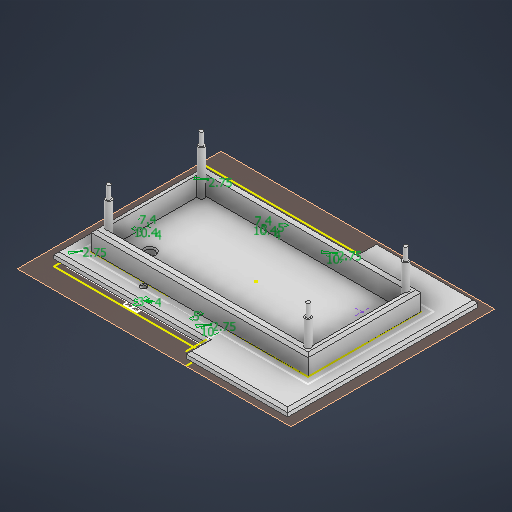
# Autodesk Inventor part: bot-buggy-body-assembly-ready-group2
Saved by Autodesk Inventor 2026.2 (Build 302298010, 298A)
## iProperties
Created: 2026-02-09
Part Number: bot-buggy-body-assembly-ready-group2
Material: Generic
Document SubType Name: Modeling
Designer: dm2166
Density: 1 g/cm^3
Appearance: Default
Mass: 226.605 g
Surface Area: 796.438 cm^2
Volume: 226.605 cm^3
Author: dm2166
Autodesk Inventor part; units mm, degrees
ref_plane "YZ Plane" through (0, 0, 0) normal (1, 0, 0) x (0, 1, 0)
ref_plane "XZ Plane" through (0, 0, 0) normal (0, 1, 0) x (-1, 0, 0)
ref_plane "XY Plane" through (0, 0, 0) normal (0, 0, 1) x (1, 0, 0)
sketch "Sketch1" plane through (0, 0, 0) normal (0, 1, 0) x (-1, 0, 0)
  line L0 (-85.5, -44.5) -> (85.5, -44.5)
  line L1 (85.5, -44.5) -> (85.5, 44.5)
  line L2 (85.5, 44.5) -> (-85.5, 44.5)
  line L3 (-85.5, 44.5) -> (-85.5, -44.5)
  line L4 (-85.5, -44.5) -> (85.5, 44.5) construction
  line L5 (85.5, -44.5) -> (-85.5, 44.5) construction
  line L6 (-81, -38.5) -> (81, -38.5)
  line L7 (81, -38.5) -> (81, 38.5)
  line L8 (81, 38.5) -> (-81, 38.5)
  line L9 (-81, 38.5) -> (-81, -38.5)
  line L10 (-81, -38.5) -> (81, 38.5) construction
  line L11 (81, -38.5) -> (-81, 38.5) construction
  line L12 (81, 38.5) -> (79.55, 38.5)
  line L13 (81, 37.05) -> (81, 38.5)
  circle A0 centre (79.55, 36.5) radius 1.45
  circle A1 centre (79.55, -36.5) radius 1.45
  circle A2 centre (-79.55, -38.5) radius 1.45
  circle A3 centre (-79.55, 38.4727) radius 1.45
  line L14 (81, -38.5) -> (81, -35.6)
  line L15 (-81, -38.5) -> (-78.1, -38.5)
  line L16 (-81, 38.5) -> (-81, 35.6)
  circle A4 centre (-79.55, 38.4727) radius 2.5
  line L17 (-95.5566, 0) -> (75.4434, 0)
  line L18 (0, 31.9167) -> (0, -57.0833)
  circle A5 centre (-79.55, -38.5) radius 2.5
  circle A6 centre (79.55, 36.5) radius 2.5
  circle A7 centre (79.55, -36.5) radius 2.5
  line L19 (140, 0) -> (-140, 0) projected
  line L20 (0, -105) -> (0, 105) projected
  line L21 (-100, 59.2475) -> (100, 59.2475)
  line L22 (100, 59.2475) -> (100, -59.2475)
  line L23 (100, -59.2475) -> (-100, -59.2475)
  line L24 (-100, -59.2475) -> (-100, 59.2475)
  line L25 (-100, 59.2475) -> (100, -59.2475) construction
  line L26 (100, 59.2475) -> (-100, -59.2475) construction
  line L27 (-100, 75) -> (-20, 75)
  line L28 (-20, 75) -> (-20, -75)
  line L29 (-20, -75) -> (-100, -75)
  line L30 (-100, -75) -> (-100, 75)
  line L31 (-100, 75) -> (-20, -75) construction
  line L32 (-20, 75) -> (-100, -75) construction
  line L33 (-79.55, 38.5) -> (-79.55, -38.5)
  line L34 (79.55, 36.5) -> (79.55, -36.5)
  line L35 (-96.0841, 75) -> (-26.0841, 75)
  line L36 (-26.0841, -75) -> (-94.0841, -75)
  point P0 (0, 0)
  point P1 (-80.9997, 38.5)
  point P2 (-81, 38.4727)
  point P3 (-81, -38.5)
  point P4 (-81, -38.5)
  point P5 (79.55, -38.5)
  point P6 (81, -36.5)
  point P7 (81, 36.5)
  point P8 (-60, 0)
  point P9 (-20, 59.2475)
  point P10 (-20, -59.2475)
  point P11 (-79.55, 0)
  point P12 (-78.1003, 38.5)
  point P13 (79.55, 0)
  dimension "d0" = 171
  dimension "d1" = 89
  dimension "d2" = 162
  dimension "d3" = 77
  dimension "d7" = 2.9
  dimension "d8" = 2.9
  dimension "d9" = 2.9
  dimension "d10" = 2.9
  dimension "d53" = 5
  dimension "d56" = 200
  dimension "d57" = 80
  dimension "d58" = 150
  dimension "d82" = 77
  dimension "d84" = 36.5
  dimension "d85" = 36.5
  constraints: 70 end point, 11 parallel, 10 midpoint, 8 centre point, 7 horizontal, 6 perpendicular, 5 point on line, 3 collinear, 3 concentric, 1 vertical, 4 other
  measures "d0" distance of L2.end L1.end
  measures "d1" distance of L1.end L0.end
  measures "d2" distance of L8.end L7.end
  measures "d3" distance of L7.end L6.end
  measures "d7" diameter of A0
  measures "d8" diameter of A1
  measures "d9" diameter of A2
  measures "d10" diameter of A3
  measures "d53" diameter of A4
  measures "d56" distance of L22.end L23.end
  measures "d57" distance of L28.end L29.end
  measures "d58" distance of L27.end L28.end
  measures "d82" distance of L33.start L33.end
  measures "d84" distance of point (79.55, 0) A1.centre
  measures "d85" distance from line of L19 A0.centre
extrude "Extrusion1" add sketch "Sketch1" along normal blind 55 contours A2 L6 | L6 L33 A2 | L8 L33 A3 | A3 L8 | A2 L33 L6 | L33 L8 A3 | A1 | A0
extrude "Extrusion2" add sketch "Sketch1" along normal blind 10 contours L28 L17 L18 L6 | L6 A5 L33 L17 L28 | L17 L33 A5 L9 | L9 A4 L33 L17 | L18 L17 L19 L34 A7 L6 | L6 A2 L33 A5 | L28 L8 L20 L18 L17 | L17 L33 A4 L8 L28 | A5 L33 A2 L9 | A7 L34 A1 L7 L6 | L18 L20 L8 A6 L34 L19 L17 | L6 L33 A2 | L8 L33 A3 | L9 A3 L33 A4 | A2 L33 L6 | L33 A3 L8 A4 | L19 L34 A6 L7 | L7 A7 L34 L19 | A7 L7 A1 L34 | L33 L8 A3 | A6 L34 A0 L7 | A1 | L8 L7 A0 L34 A6 | A0
extrude "Extrusion3" add sketch "Sketch1" along normal blind 25 contours L3 L17 L9 A5 L6 L28 L0 | L28 L6 L18 L0 | L3 L2 L28 L8 A4 L9 L17 | L18 L6 A7 L7 L19 L1 L0 | A5 L9 A2 L6 | L2 L20 L8 L28 | L19 L7 A6 L8 L20 L2 L1 | L6 L7 A7 | A2 L6 | A4 L8 A3 L9 | A3 L8 | L7 L8 A6
chamfer "Chamfer1" distance 2 angle 45 4 edges at (0, 25, 44.5) (85.5, 25, 0) (0, 25, -44.5) (-85.5, 25, 0)
extrude "Extrusion11" add sketch "Sketch1" along normal blind 45 contours A5 L9 A2 L6 | L6 A2 L33 A5 | A5 L33 A2 L9 | A7 L34 A1 L7 L6 | L6 L7 A7 | A2 L6 | L6 L33 A2 | L8 L33 A3 | A4 L8 A3 L9 | A3 L8 | L9 A3 L33 A4 | A2 L33 L6 | L33 A3 L8 A4 | A7 L7 A1 L34 | L33 L8 A3 | A6 L34 A0 L7 | L7 L8 A6 | A1 | L8 L7 A0 L34 A6 | A0
extrude "Extrusion12" add sketch "Sketch1" along normal blind 10 contours L0 L28 L23 L24 L19 L17 L3 | L0 L18 L20 L23 L28 | L17 L19 L24 L21 L28 L2 L3 | L0 L1 L19 L22 L23 L20 L18 | L28 L29 L30 L23 | L28 L21 L20 L2 | L1 L2 L20 L21 L22 L19 | L21 L30 L27 L28
chamfer "Chamfer2" distance 2 angle 45 8 edges at (100, 10, 0) (60, 10, 75) (20, 10, 67.1238) (60, 10, -75) (20, 10, -67.1238) (-40, 10, -59.2475) (-40, 10, 59.2475) (-100, 10, 0)
sketch "Sketch4" plane through (0, 0, 0) normal (0, -1, 0) x (1, 0, 0)
  circle A0 centre (-11.2675, 0) radius 2 projected
  circle A1 centre (-71.2675, 0) radius 2 projected
  circle A2 centre (-41.2675, 30) radius 2 projected
  circle A3 centre (-11.2675, 0) radius 1.9
  circle A4 centre (-71.2675, 0) radius 1.9
  circle A5 centre (-41.2675, 30) radius 1.9
  point P0 (0, 0)
  dimension "d64" = 3.8
  constraints: 3 centre point, 3 coincident, 2 equal radius
  measures "d64" diameter of A5
extrude "Extrusion13" add sketch "Sketch4" along normal blind 10 contours A3 | A4 | A5
sketch "Sketch7" plane through (0, 0, 0) normal (0, -1, 0) x (1, 0, 0)
  line L0 (20, -59.2475) -> (-100, -59.2475) projected
  line L1 (20, -75) -> (20, -59.2475) projected
  line L2 (100, -75) -> (20, -75) projected
  line L3 (100, 75) -> (100, -75) projected
  line L4 (20, 75) -> (100, 75) projected
  line L5 (20, 59.2475) -> (20, 75) projected
  line L6 (-100, 59.2475) -> (20, 59.2475) projected
  line L7 (-100, -59.2475) -> (-100, 59.2475) projected
  line L8 (-95, -54.2475) -> (25, -54.2475)
  line L9 (25, -54.2475) -> (25, -70)
  line L10 (25, -70) -> (95, -70)
  line L11 (95, -70) -> (95, 70)
  line L12 (95, 70) -> (25, 70)
  line L13 (25, 70) -> (25, 54.2475)
  line L14 (25, 54.2475) -> (-95, 54.2475)
  line L15 (-95, 54.2475) -> (-95, -54.2475)
  line L16 (-90, -49.2475) -> (30, -49.2475)
  line L17 (30, -49.2475) -> (30, -65)
  line L18 (30, -65) -> (90, -65)
  line L19 (90, -65) -> (90, 65)
  line L20 (90, 65) -> (30, 65)
  line L21 (30, 65) -> (30, 49.2475)
  line L22 (30, 49.2475) -> (-90, 49.2475)
  line L23 (-90, 49.2475) -> (-90, -49.2475)
  circle A0 centre (25, -70) radius 2
  circle A1 centre (25, 70) radius 2
  circle A2 centre (-41.2675, 0) radius 44 projected
  line L24 (-41.2675, -59.2475) -> (-41.2675, 59.2475)
  line L25 (17.4651, 0) -> (-100, 0)
  point P0 (0, 0)
  dimension "d86" = 5
  dimension "d87" = 10
  dimension "d88" = 4
  dimension "d89" = 4
  constraints: 36 end point, 3 midpoint, 2 centre point, 2 coincident, 1 perpendicular, 1 point on line, 14 other
  measures "d86" distance between parallel lines of L0 L8
  measures "d87" distance between parallel lines of L0 L16
  measures "d88" diameter of A0
  measures "d89" diameter of A1
extrude "Extrusion15" add sketch "Sketch7" along normal blind 10 contours A0 L10 L9 | L9 L10 A0 | A1 L12 L13 | L13 L12 A1
fillet "Fillet16" radius 1 1 edges at (23, -10, -70)
fillet "Fillet17" radius 1 1 edges at (23, 0, -70)
fillet "Fillet18" radius 1 1 edges at (23, 0, 70)
fillet "Fillet19" radius 1 1 edges at (23, -10, 70)
sketch "Sketch9" plane through (0, 0, 0) normal (0, -1, 0) x (1, 0, 0)
  line L0 (-100, 59.2475) -> (20, 59.2475) projected
  line L1 (20, -75) -> (20, 75) projected
  line L2 (20, -59.2475) -> (-100, -59.2475) projected
  line L3 (-100, -59.2475) -> (-100, 59.2475) projected
  circle A0 centre (-41.2675, 0) radius 44 projected
  line L4 (-41.2675, -59.2475) -> (-41.2675, 59.2475)
  line L5 (17.4651, 0) -> (-100, 0)
  line L6 (20, -54.2475) -> (-95, -54.2475)
  line L7 (-95, -54.2475) -> (-95, 54.2475)
  line L8 (-95, 54.2475) -> (20, 54.2475)
  line L9 (-36.0675, -57.9475) -> (-46.4675, -57.9475)
  line L10 (-46.4675, -57.9475) -> (-46.4675, -50.5475)
  line L11 (-46.4675, -50.5475) -> (-36.0675, -50.5475)
  line L12 (-36.0675, -50.5475) -> (-36.0675, -57.9475)
  line L13 (-36.0675, -57.9475) -> (-46.4675, -50.5475) construction
  line L14 (-46.4675, -57.9475) -> (-36.0675, -50.5475) construction
  line L15 (-36.0675, 57.9475) -> (-46.4675, 57.9475)
  line L16 (-46.4675, 57.9475) -> (-46.4675, 50.5475)
  line L17 (-46.4675, 50.5475) -> (-36.0675, 50.5475)
  line L18 (-36.0675, 50.5475) -> (-36.0675, 57.9475)
  line L19 (-36.0675, 57.9475) -> (-46.4675, 50.5475) construction
  line L20 (-46.4675, 57.9475) -> (-36.0675, 50.5475) construction
  line L21 (-36.0675, -50.5475) -> (-46.4675, -50.5475)
  line L22 (-98.7, 5.2) -> (-91.3, 5.2)
  line L23 (-91.3, 5.2) -> (-91.3, -5.2)
  line L24 (-91.3, -5.2) -> (-98.7, -5.2)
  line L25 (-98.7, -5.2) -> (-98.7, 5.2)
  line L26 (-98.7, 5.2) -> (-91.3, -5.2) construction
  line L27 (-91.3, 5.2) -> (-98.7, -5.2) construction
  line L28 (-91.3, 0) -> (-88.3, 0)
  circle A1 centre (-88.3, 0) radius 2
  line L29 (-41.2675, -50.5475) -> (-41.2675, -47.5475)
  line L30 (-41.2675, 50.5475) -> (-41.2675, 47.5475)
  circle A2 centre (-41.2675, 47.5475) radius 2
  circle A3 centre (-41.2675, -47.5475) radius 2
  point P0 (0, 0)
  point P1 (-41.2675, -54.2475)
  point P2 (-41.2675, 54.2475)
  point P3 (-95, 0)
  dimension "d99" = 5
  dimension "d100" = 10.4
  dimension "d101" = 7.4
  dimension "d103" = 7.4
  dimension "d104" = 10.4
  dimension "d110" = 3
  dimension "d111" = 4
  dimension "d112" = 3
  dimension "d115" = 3
  dimension "d116" = 4
  dimension "d117" = 4
  constraints: 54 end point, 11 midpoint, 6 point on line, 5 symmetric about line, 4 parallel, 3 centre point, 3 coincident, 3 horizontal, 3 perpendicular, 2 other
  measures "d99" distance between parallel lines of L2 L6
  measures "d100" distance of L10.end L11.end
  measures "d101" distance of L9.end L10.end
  measures "d103" distance of L23.end L24.end
  measures "d104" distance of L22.end L23.end
  measures "d110" distance of L28.start L28.end
  measures "d111" diameter of A1
  measures "d112" distance of L29.start L29.end
  measures "d115" distance of L30.start L30.end
  measures "d116" diameter of A2
  measures "d117" diameter of A3
extrude "Extrusion17" cut sketch "Sketch9" against normal blind 8.5 contours L15 L18 L8 L4 | L4 L8 L16 L15 | L25 L22 L7 L5 | L5 L7 L24 L25 | L8 L18 L17 L4 | L4 L17 L16 L8 | L7 L22 L23 L5 | L5 L23 L24 L7 | L9 L10 L6 L4 | L4 L6 L12 L9 | L6 L4 L11 L12 | L6 L10 L11 L4
fillet "Fillet20" radius 1 6 edges at (-95, 8.5, 5.2) (-95, 8.5, -5.2) (-46.4675, 8.5, -54.2475) (-36.0675, 8.5, -54.2475) (-36.0675, 8.5, 54.2475) (-46.4675, 8.5, 54.2475)
sketch "Sketch10" plane through (0, 0, 0) normal (0, -1, 0) x (1, 0, 0)
  circle A0 centre (-41.2675, 47.5475) radius 2 projected
  circle A1 centre (-41.2675, -47.5475) radius 2 projected
  circle A2 centre (-88.3, 0) radius 2 projected
  point P0 (0, 0)
extrude "Extrusion18" cut sketch "Sketch10" against normal blind 15
sketch "Sketch11" plane through (0, 10, 0) normal (0, 1, 0) x (1, 0, 0)
  circle A0 centre (-168.2379, -151.522) radius 7.5
  circle A1 centre (-62.4807, -21.2132) radius 7.5 projected
  circle A2 centre (-62.4807, -21.2132) radius 3.75
  point P0 (0, 0)
  dimension "d134" = 7.5
  constraints: 2 centre point, 1 coincident
  measures "d134" diameter of A2
sketch "Sketch12" plane through (0, 10, 0) normal (0, 1, 0) x (1, 0, 0)
  line L0 (-85.5, -44.5) -> (85.5, -44.5) projected
  line L1 (-85.5, 44.5) -> (-85.5, -44.5) projected
  line L2 (85.5, 44.5) -> (-85.5, 44.5) projected
  line L3 (85.5, -44.5) -> (85.5, 44.5) projected
  line L4 (90.5, -49.5) -> (-90.5, -49.5)
  line L5 (-90.5, -49.5) -> (-90.5, 49.5)
  line L6 (-90.5, 49.5) -> (90.5, 49.5)
  line L7 (90.5, 49.5) -> (90.5, -49.5)
  circle A0 centre (-90.5, 49.5) radius 1.375
  circle A1 centre (-90.5, -49.5) radius 1.375
  line L8 (20, -59.2475) -> (20, -75) projected
  line L9 (20, -59.2475) -> (20, -44.5)
  line L10 (20, 59.2475) -> (-100, 59.2475) projected
  line L11 (20, 59.2475) -> (20, 44.5)
  line L12 (20, -49.5) -> (10, -49.5)
  line L13 (20, 49.5) -> (10, 49.5)
  circle A2 centre (10, -49.5) radius 1.375
  circle A3 centre (10, 49.5) radius 1.375
  point P0 (0, 0)
  point P1 (62.481, 21.213)
  dimension "d120" = 5
  dimension "d123" = 2.75
  dimension "d124" = 2.75
  dimension "d127" = 10
  dimension "d128" = 10
  dimension "d129" = 2.75
  dimension "d130" = 2.75
  constraints: 16 end point, 9 point on line, 4 centre point, 4 coincident, 1 perpendicular, 3 other
  measures "d120" distance between parallel lines of L0 L4
  measures "d123" diameter of A0
  measures "d124" diameter of A1
  measures "d127" distance of L12.start L12.end
  measures "d128" distance of L13.start L13.end
  measures "d129" diameter of A2
  measures "d130" diameter of A3
extrude "Extrusion19" cut sketch "Sketch12" against normal blind 14 contours A1 L5 L4 | L4 L5 A1 | A0 L5 L6 | L6 L5 A0
extrude "Extrusion20" cut sketch "Sketch12" against normal blind 14 contours A2 L4 | L4 A2 | A3 L6 | L6 A3
fillet "Fillet21" radius 1 6 edges at (-73.1675, 0, 0) (-73.1675, -10, 0) (-43.1675, -10, 30) (-43.1675, 0, 30) (-13.1675, 0, 0) (-13.1675, -10, 0)
extrude "Extrusion21" cut sketch "Sketch11" against normal blind 14 contours A2
fillet "Fillet22" radius 1 2 edges at (-66.2307, 0, 21.2132) (-66.2307, 10, 21.2132)
chamfer "Chamfer4" distance 1 angle 45 4 edges at (8.625, 0, 49.5) (8.625, 0, -49.5) (-91.875, 0, -49.5) (-91.875, 0, 49.5)
fillet "Fillet23" radius 0.5 6 edges at (-90.3, 0, 0) (-43.2675, 0, -47.5475) (-43.2675, 0, 47.5475) (-90.3, 10, 0) (-43.2675, 10, 47.5475) (-43.2675, 10, -47.5475)
ref_plane "Work Plane3" through (0, 5, 0) normal (0, 1, 0) x (1, 0, 0)
split "Split1" plane through (0, 5, 0) removes the side toward (0, -1, 0)
body "Solid1"
